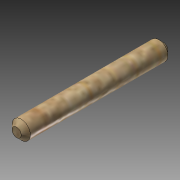
# Autodesk Inventor part: 97195A419
Saved by Autodesk Inventor 2015 SP2 (Build 190223200, 223)
## iProperties
Company: Showman Fabricators
Created: 2016-05-10
Part Number: 97195A419
Material: LUMBER WHITE PINE D SELECT
Document SubType Name: Modeling
Designer: Josh
Density: 0.480551 g/cm^3
Sheet Metal Rule: Default
Appearance: Pine - Coarse
Description: Wood Dowel Pin, 1/4" Diameter, 2" Length
Vendor: MCMASTER-CARR
CNC: False
Author: Josh
Autodesk Inventor part; units mm, degrees
ref_plane "YZ Plane" through (0, 0, 0) normal (1, 0, 0) x (0, 1, 0)
sketch "CORNER RELIEF 3-8 BIT" plane through (0, 0, 0) normal (0, 0, 1) x (1, 0, 0)
  circle A0 centre (0, 0) radius 5.08
  point P0 (-5.08, 0)
  point P1 (0, 5.08)
  point P2 (5.08, 0)
  point P3 (0, -5.08)
  dimension "d5" = 3.175
  dimension "Thickness" = 3.048
  dimension "d0" = 10.16
  measures "d0" diameter of A0
sketch "Sketch2" plane through (0, 0, 0) normal (0, 0, 1) x (1, 0, 0)
  circle A0 centre (0, 0) radius 3.175
  dimension "d1" = 6.35
  constraints: 1 centre point, 1 coincident
  measures "d1" diameter of A0
extrude "Extrusion1" add sketch "Sketch2" along normal mid plane 50.8
chamfer "Chamfer1" distance 1.5875 angle 45 2 edges at (-3.175, 0, 25.4) (-3.175, 0, -25.4)
ref_plane "Work Plane1" through (0, 0, -11.1125) normal (0, 0, 1) x (1, 0, 0)
ref_plane "Work Plane2" through (0, 0, 11.1125) normal (0, 0, 1) x (1, 0, 0)
equation "\"PLY_1_2_THICK\" = 11.90752"
equation "\"PLY_3_4_THICK\" = 18.25752"
equation "\"WIG_WD_1_4_THICK\" = 4.7625"
equation "\"WIG_WD_3_8_THICK\" = 7.9375"
equation "\"MDF_1_2_THICK\" = 12"
equation "\"MDF_3_4_THICK\" = 18"
equation "\"BendRadius\" = Thickness"
equation "\"BendReliefWidth\" = Thickness"
equation "\"BendReliefDepth\" = 0.5 * Thickness"
equation "\"CornerReliefSize\" = 4 * Thickness"
equation "\"MinimumRemnant\" = 2 * Thickness"
equation "\"TransitionRadius\" = BendRadius"
equation "\"JacobiRadiusSize\" = BendRadius"
equation "\"GapSize\" = Thickness"
body "Solid1"
